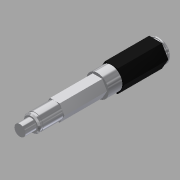
# Autodesk Inventor part: Primary Shaft
Saved by Autodesk Inventor 2013 (Build 170138000, 138)
## iProperties
Created: 2013-07-09
Part Number: Primary Shaft
Material: Generic
Document SubType Name: Modeling
Designer: mvarma
Density: 1 g/cm^3
Author: mvarma
Autodesk Inventor part; units mm, degrees
ref_plane "YZ Plane" through (0, 0, 0) normal (1, 0, 0) x (0, 1, 0)
ref_plane "XZ Plane" through (0, 0, 0) normal (0, 1, 0) x (-1, 0, 0)
ref_plane "XY Plane" through (0, 0, 0) normal (0, 0, 1) x (1, 0, 0)
sketch "Sketch1" plane through (0, 0, 0) normal (0, 0, 1) x (1, 0, 0)
  line L0 (-5.4993, 0) -> (-2.7496, 4.7625)
  line L1 (-2.7496, 4.7625) -> (2.7496, 4.7625)
  line L2 (2.7496, 4.7625) -> (5.4993, 0)
  line L3 (5.4993, 0) -> (2.7496, -4.7625)
  line L4 (2.7496, -4.7625) -> (-2.7496, -4.7625)
  line L5 (-2.7496, -4.7625) -> (-5.4993, 0)
  point P0 (0, 0)
  point P1 (0, 0)
  dimension "d58" = 1.5875
  dimension "d59" = 0
  dimension "d0" = 9.525
  constraints: 12 end point, 1 coincident, 1 horizontal, 13 other
  measures "d0" distance between parallel lines of L4 L1
extrude "3/8 Hex" add sketch "Sketch1" along normal blind 24.511
sketch "Sketch2" plane through (0, 0, 24.511) normal (0, 0, 1) x (1, 0, 0)
  circle A0 centre (0, 0) radius 4.7625
  dimension "d3" = 9.525
  constraints: 1 centre point, 1 coincident
  measures "d3" diameter of A0
extrude "3/8 Round" add sketch "Sketch2" along normal blind 11.3347
sketch "Sketch3" plane through (0, 0, 35.8458) normal (0, 0, 1) x (1, 0, 0)
  circle A0 centre (0, 0) radius 4.7625 projected
  circle A1 centre (0, 0) radius 3.175
  dimension "d6" = 6.35
  constraints: 1 centre point, 1 coincident
  measures "d6" diameter of A1
extrude "Extrusion3" add sketch "Sketch3" along normal blind 8.6741 contours A1
sketch "Sketch7" plane through (0, 0, 0) normal (0, 0, -1) x (-1, 0, 0)
  circle A0 centre (0, 0) radius 6.35
  dimension "d18" = 12.7
  constraints: 1 centre point, 1 coincident
  measures "d18" diameter of A0
extrude "1/2 Round" add sketch "Sketch7" along normal blind 7.9375
sketch "Sketch8" plane through (0, 0, -7.9375) normal (0, 0, -1) x (-1, 0, 0)
  circle A0 centre (0, 0) radius 6.35 projected
  line L0 (-7.3323, 0) -> (-3.6662, 6.35)
  line L1 (-3.6662, 6.35) -> (3.6662, 6.35)
  line L2 (3.6662, 6.35) -> (7.3323, 0)
  line L3 (7.3323, 0) -> (3.6662, -6.35)
  line L4 (3.6662, -6.35) -> (-3.6662, -6.35)
  line L5 (-3.6662, -6.35) -> (-7.3323, 0)
  dimension "d21" = 12.7
  constraints: 12 end point, 1 coincident, 1 horizontal, 13 other
  measures "d21" distance between parallel lines of L4 L1
extrude "1/2 Hex" add sketch "Sketch8" along normal blind 25.4
sketch "Sketch12" plane through (0, 0, -33.3375) normal (0, 0, -1) x (-1, 0, 0)
  circle A0 centre (0, 0) radius 5.9436
  dimension "d41" = 11.8872
  constraints: 1 centre point, 1 coincident
  measures "d41" diameter of A0
extrude "Spring Clip Groove" add sketch "Sketch12" along normal blind 0.9906
sketch "Sketch13" plane through (0, 0, -34.3281) normal (0, 0, -1) x (-1, 0, 0)
  circle A0 centre (0, 0) radius 5.9436 projected
  circle A1 centre (0, 0) radius 6.35
  dimension "d45" = 12.7
  constraints: 1 centre point, 1 coincident
  measures "d45" diameter of A1
extrude "Spring Clip" add sketch "Sketch13" along normal blind 1.5875 contours A0 | A1
chamfer "Chamfer2" distance 0.7937 angle 45 1 edges at (6.35, 0, -35.9156)
sketch "Sketch14" plane through (0, 0, 35.8458) normal (0, 0, 1) x (1, 0, 0)
  circle A0 centre (0, 0) radius 3.175 projected
  circle A1 centre (0, 0) radius 4.7625 projected
  circle A2 centre (0, 0) radius 4.4704
  dimension "d52" = 8.9408
  constraints: 1 centre point, 1 coincident
  measures "d52" diameter of A2
extrude "3/8 Spring Clip Groove" add sketch "Sketch14" along normal blind 0.7366 contours A2
sketch "Sketch15" plane through (0, 0, 36.5823) normal (0, 0, 1) x (1, 0, 0)
  circle A0 centre (0, 0) radius 3.175 projected
  circle A1 centre (0, 0) radius 4.4704 projected
  circle A2 centre (0, 0) radius 4.7625
  dimension "d56" = 9.525
  constraints: 1 centre point, 1 coincident
  measures "d56" diameter of A2
extrude "Extrusion14" add sketch "Sketch15" along normal blind 1.5875 contours A1 | A2
chamfer "Chamfer3" distance 0.7937 angle 45 1 edges at (-4.7625, 0, 38.1698)
body "Solid1"
